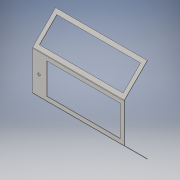
# Autodesk Inventor part: door
Saved by Autodesk Inventor 2016 (Build 200138000, 138)
## iProperties
Created: 2017-08-29
Part Number: door
Material: Generic
Document SubType Name: Sheet Metal
Designer: m207653
Density: 1 g/cm^3
Sheet Metal Rule: Default_mm
Appearance: Default
Author: m207653
Autodesk Inventor part; units mm, degrees
ref_plane "YZ Plane" through (0, 0, 0) normal (1, 0, 0) x (0, 1, 0)
ref_plane "XZ Plane" through (0, 0, 0) normal (0, 1, 0) x (-1, 0, 0)
ref_plane "XY Plane" through (0, 0, 0) normal (0, 0, 1) x (1, 0, 0)
sketch "Sketch1" plane through (0, 0, 0) normal (0, 1, 0) x (-1, 0, 0)
  line L0 (0, 0) -> (-700, 0)
  line L1 (-700, 0) -> (-700, 300)
  line L2 (-700, 300) -> (0, 300)
  line L3 (0, 300) -> (0, 0)
  dimension "d0" = 700
  dimension "d1" = 300
  measures "d0" distance of L0.start L0.end
  measures "d1" distance of L0.end L1.end
extrude "Plate1" add sketch "Sketch1" along normal blind 3
sketch "Sketch2" plane through (0, 2.1213, 297.8787) normal (0, -0.7071068, 0.7071068) x (-1, 0, 0)
  line L0 (-700, 0) -> (0, 0)
  line L1 (0, 0) -> (0, 250)
  line L2 (0, 250) -> (-700, 250)
  line L3 (-700, 250) -> (-700, 0)
  constraints: 6 end point, 1 horizontal, 1 perpendicular, 1 vertical
edge flange "Flange1" height 250 angle -45 thickness 3 bend radius 3 thickness toward (0, -0.7071068, 0.7071068) relief straight relief width 3 relief depth 1.5 edges at (350, 0, 300) wall of the first edge with corners at (700, 2.1213, 297.8787) (0, 2.1213, 297.8787) (0, 178.898, 474.6554) (700, 178.898, 474.6554)
bend "Bend1"
corner "Corner1"
sketch "Sketch3" plane through (700, 2.1213, 2.1213) normal (0, -0.7071068, -0.7071068) x (-1, 0, 0)
  line L0 (700, 0) -> (0, 0)
  line L1 (0, 0) -> (0, -250)
  line L2 (0, -250) -> (700, -250)
  line L3 (700, -250) -> (700, 0)
  constraints: 6 end point, 1 horizontal, 1 perpendicular, 1 vertical
edge flange "Flange2" height 250 angle -45 thickness 3 bend radius 3 thickness toward (0, -0.7071068, -0.7071068) relief straight relief width 3 relief depth 1.5 edges at (350, 0, 0) wall of the first edge with corners at (0, 2.1213, 2.1213) (700, 2.1213, 2.1213) (700, 178.898, -174.6554) (0, 178.898, -174.6554)
bend "Bend2"
corner "Corner2"
sketch "Sketch4" plane through (0, 0, 0) normal (0, -1, 0) x (1, 0, 0)
  circle A0 centre (50, 147.5147) radius 10
  line L0 (0, 297.5147) -> (0, 2.4853) projected
  line L1 (700, 297.5147) -> (0, 297.5147) projected
  point P0 (0, 0)
  dimension "d23" = 20
  dimension "d24" = 50
  dimension "d25" = 150
  constraints: 1 centre point
  measures "d23" diameter of A0
  measures "d24" distance from line of L0 A0.centre
  measures "d25" distance from line of L1 A0.centre
hole "Hole1" at (50, 0, 147.5147) direction (0, 1, 0) diameter 20 end through all
sketch "Sketch5" plane through (0, 176.7767, 476.7767) normal (0, -0.7071068, 0.7071068) x (1, 0, 0)
  line L0 (30, -30) -> (670, -30)
  line L1 (670, -30) -> (670, -217.5147)
  line L2 (670, -217.5147) -> (30, -217.5147)
  line L3 (30, -217.5147) -> (30, -30)
  line L4 (700, 0) -> (0, 0) projected
  line L5 (0, -247.5147) -> (0, 0) projected
  line L6 (0, -247.5147) -> (700, -247.5147) projected
  line L7 (700, -247.5147) -> (700, 0) projected
  point P0 (0, -462.132)
  dimension "d33" = 30
  dimension "d34" = 30
  dimension "d35" = 30
  dimension "d36" = 30
  constraints: 8 end point, 2 parallel, 1 horizontal, 1 perpendicular
  measures "d33" distance between parallel lines of L4 L0
  measures "d34" distance between parallel lines of L5 L3
  measures "d35" distance between parallel lines of L6 L2
  measures "d36" distance between parallel lines of L7 L1
extrude "Cut1" cut sketch "Sketch5" against normal blind 3 contours L0 L1 L2 L3
sketch "Sketch6" plane through (700, 176.7767, -176.7767) normal (0, -0.7071068, -0.7071068) x (-1, 0, 0)
  line L0 (30, -30) -> (670, -30)
  line L1 (670, -30) -> (670, -217.5147)
  line L2 (670, -217.5147) -> (30, -217.5147)
  line L3 (30, -217.5147) -> (30, -30)
  line L4 (700, 0) -> (0, 0)
  line L5 (0, -247.5147) -> (0, 0)
  line L6 (0, -247.5147) -> (700, -247.5147)
  line L7 (700, -247.5147) -> (700, 0)
  point P0 (700, -250)
  point P1 (0, -462.132)
  dimension "d39" = 30
  dimension "d40" = 30
  dimension "d41" = 30
  dimension "d42" = 30
  constraints: 16 end point, 2 parallel, 1 horizontal, 1 perpendicular
  measures "d39" distance between parallel lines of L4 L0
  measures "d40" distance between parallel lines of L5 L3
  measures "d41" distance between parallel lines of L6 L2
  measures "d42" distance between parallel lines of L7 L1
extrude "Cut2" cut sketch "Sketch6" against normal blind 3 contours L0 L1 L2 L3
sketch "Sketch7" plane through (0, 0, 0) normal (0, -1, 0) x (1, 0, 0)
  line L0 (110, 267.5147) -> (670, 267.5147)
  line L1 (670, 267.5147) -> (670, 32.4853)
  line L2 (670, 32.4853) -> (110, 32.4853)
  line L3 (110, 32.4853) -> (110, 267.5147)
  line L4 (0, 297.5147) -> (700, 297.5147) projected
  line L5 (0, 2.4853) -> (700, 2.4853) projected
  line L6 (700, 2.4853) -> (700, 297.5147) projected
  circle A0 centre (50, 147.5147) radius 10 projected
  point P0 (0, 0)
  dimension "d45" = 30
  dimension "d46" = 30
  dimension "d47" = 30
  dimension "d48" = 60
  constraints: 8 end point, 2 parallel, 1 horizontal, 1 perpendicular
  measures "d45" distance between parallel lines of L4 L0
  measures "d46" distance between parallel lines of L5 L2
  measures "d47" distance between parallel lines of L6 L1
  measures "d48" distance from line of L3 A0.centre
extrude "Cut3" cut sketch "Sketch7" against normal blind 3 contours L0 L1 L2 L3
equation "\"d31\" = Thickness"
equation "\"d37\" = Thickness"
equation "\"d43\" = Thickness"
equation "\"d49\" = Thickness"
equation "\"d3\" = BendReliefWidth"
equation "\"d4\" = BendReliefDepth"
equation "\"d5\" = MinimumRemnant"
equation "\"d6\" = BendRadius"
equation "\"d9\" = BendRadius"
equation "\"d10\" = CornerReliefSize"
equation "\"d11\" = GapSize"
equation "\"d12\" = JacobiRadiusSize"
equation "\"d13\" = BendReliefWidth"
equation "\"d14\" = BendReliefDepth"
equation "\"d15\" = MinimumRemnant"
equation "\"d16\" = BendRadius"
equation "\"d19\" = BendRadius"
equation "\"d20\" = CornerReliefSize"
equation "\"d21\" = GapSize"
equation "\"d22\" = JacobiRadiusSize"
equation "\"BendRadius\" = Thickness"
equation "\"BendReliefWidth\" = Thickness"
equation "\"BendReliefDepth\" = 0.5 * Thickness"
equation "\"CornerReliefSize\" = 4 * Thickness"
equation "\"MinimumRemnant\" = 2 * Thickness"
equation "\"TransitionRadius\" = BendRadius"
equation "\"JacobiRadiusSize\" = BendRadius"
equation "\"GapSize\" = Thickness"
equation "\"d2\" = BendRadius"
equation "\"Thickness\" = 3"
body "Solid1"
